Autodesk Inventor part; units mm, degrees
(part 3 of 3)
  line L2014 (13.025, -25.6738) -> (12.925, -25.6738)
  line L2015 (12.9, -26.05) -> (12.8, -26.05)
  line L2016 (12.65, -26.05) -> (12.55, -26.05)
  line L2017 (12.9, -26.35) -> (12.9, -26.05)
  line L2018 (12.8, -26.05) -> (12.8, -26.35)
  line L2019 (12.65, -26.35) -> (12.65, -26.05)
  line L2020 (12.55, -26.05) -> (12.55, -26.35)
  line L2021 (13.4, -26.35) -> (13.4, -26.05)
  line L2022 (13.3, -26.35) -> (13.4, -26.35)
  line L2023 (13.3, -26.05) -> (13.3, -26.35)
  line L2024 (13.15, -26.05) -> (13.05, -26.05)
  line L2025 (13.15, -26.35) -> (13.15, -26.05)
  line L2026 (13.05, -26.05) -> (13.05, -26.35)
  line L2027 (12.8, -26.35) -> (12.9, -26.35)
  line L2028 (12.55, -26.35) -> (12.65, -26.35)
  line L2029 (13.275, -25.9738) -> (13.275, -25.6738)
  line L2030 (13.425, -25.6738) -> (13.425, -25.9738)
  line L2031 (13.525, -25.6738) -> (13.425, -25.6738)
  line L2032 (13.425, -25.9738) -> (13.525, -25.9738)
  line L2033 (13.525, -25.9738) -> (13.525, -25.6738)
  line L2034 (13.675, -25.6738) -> (13.675, -25.9738)
  line L2035 (13.65, -26.05) -> (13.55, -26.05)
  line L2036 (13.775, -25.6738) -> (13.675, -25.6738)
  line L2037 (13.775, -25.9738) -> (13.775, -25.6738)
  line L2038 (13.675, -25.9738) -> (13.775, -25.9738)
  line L2039 (13.4, -26.05) -> (13.3, -26.05)
  line L2040 (13.925, -25.9738) -> (14.025, -25.9738)
  line L2041 (13.925, -25.6738) -> (13.925, -25.9738)
  line L2042 (14.025, -25.9738) -> (14.025, -25.6738)
  line L2043 (14.025, -25.6738) -> (13.925, -25.6738)
  line L2044 (14.425, -25.9738) -> (14.525, -25.9738)
  line L2045 (14.175, -25.9738) -> (14.275, -25.9738)
  line L2046 (14.525, -25.9738) -> (14.525, -25.6738)
  line L2047 (14.275, -25.9738) -> (14.275, -25.6738)
  line L2048 (14.175, -25.6738) -> (14.175, -25.9738)
  line L2049 (14.425, -25.6738) -> (14.425, -25.9738)
  line L2050 (14.525, -25.6738) -> (14.425, -25.6738)
  line L2051 (14.275, -25.6738) -> (14.175, -25.6738)
  line L2052 (14.05, -26.05) -> (14.05, -26.35)
  line L2053 (14.15, -26.05) -> (14.05, -26.05)
  line L2054 (14.05, -26.35) -> (14.15, -26.35)
  line L2055 (14.15, -26.35) -> (14.15, -26.05)
  line L2056 (14.3, -26.05) -> (14.3, -26.35)
  line L2057 (14.4, -26.05) -> (14.3, -26.05)
  line L2058 (14.3, -26.35) -> (14.4, -26.35)
  line L2059 (14.4, -26.35) -> (14.4, -26.05)
  line L2060 (14.55, -26.05) -> (14.55, -26.35)
  line L2061 (13.9, -26.05) -> (13.8, -26.05)
  line L2062 (13.55, -26.05) -> (13.55, -26.35)
  line L2063 (13.55, -26.35) -> (13.65, -26.35)
  line L2064 (13.65, -26.35) -> (13.65, -26.05)
  line L2065 (13.8, -26.05) -> (13.8, -26.35)
  line L2066 (13.9, -26.35) -> (13.9, -26.05)
  line L2067 (13.8, -26.35) -> (13.9, -26.35)
  line L2068 (15.175, -25.6738) -> (15.175, -25.9738)
  line L2069 (15.175, -25.9738) -> (15.275, -25.9738)
  line L2070 (15.275, -25.6738) -> (15.175, -25.6738)
  line L2071 (15.275, -25.9738) -> (15.275, -25.6738)
  line L2072 (15.425, -25.6738) -> (15.425, -25.9738)
  line L2073 (15.525, -25.9738) -> (15.525, -25.6738)
  line L2074 (15.525, -25.6738) -> (15.425, -25.6738)
  line L2075 (15.675, -25.6738) -> (15.675, -25.9738)
  line L2076 (15.775, -25.6738) -> (15.675, -25.6738)
  line L2077 (15.775, -25.9738) -> (15.775, -25.6738)
  line L2078 (15.675, -25.9738) -> (15.775, -25.9738)
  line L2079 (15.425, -25.9738) -> (15.525, -25.9738)
  line L2080 (15.4, -26.05) -> (15.3, -26.05)
  line L2081 (15.65, -26.05) -> (15.55, -26.05)
  line L2082 (15.15, -26.05) -> (15.05, -26.05)
  line L2083 (15.55, -26.35) -> (15.65, -26.35)
  line L2084 (15.65, -26.35) -> (15.65, -26.05)
  line L2085 (15.55, -26.05) -> (15.55, -26.35)
  line L2086 (15.4, -26.35) -> (15.4, -26.05)
  line L2087 (15.3, -26.35) -> (15.4, -26.35)
  line L2088 (15.3, -26.05) -> (15.3, -26.35)
  line L2089 (15.15, -26.35) -> (15.15, -26.05)
  line L2090 (15.05, -26.05) -> (15.05, -26.35)
  line L2091 (15.05, -26.35) -> (15.15, -26.35)
  line L2092 (18.925, -25.6738) -> (18.925, -25.9738)
  line L2093 (18.925, -25.9738) -> (19.025, -25.9738)
  line L2094 (19.025, -25.6738) -> (18.925, -25.6738)
  line L2095 (19.175, -25.6738) -> (19.175, -25.9738)
  line L2096 (19.175, -25.9738) -> (19.275, -25.9738)
  line L2097 (19.275, -25.9738) -> (19.275, -25.6738)
  line L2098 (19.275, -25.6738) -> (19.175, -25.6738)
  line L2099 (19.425, -25.6738) -> (19.425, -25.9738)
  line L2100 (19.425, -25.9738) -> (19.525, -25.9738)
  line L2101 (19.525, -25.9738) -> (19.525, -25.6738)
  line L2102 (19.525, -25.6738) -> (19.425, -25.6738)
  line L2103 (19.025, -25.9738) -> (19.025, -25.6738)
  line L2104 (20.4, -26.05) -> (20.3, -26.05)
  line L2105 (20.425, -25.6738) -> (20.425, -25.9738)
  line L2106 (20.525, -25.9738) -> (20.525, -25.6738)
  line L2107 (20.525, -25.6738) -> (20.425, -25.6738)
  line L2108 (20.425, -25.9738) -> (20.525, -25.9738)
  line L2109 (20.675, -25.6738) -> (20.675, -25.9738)
  line L2110 (20.675, -25.9738) -> (20.775, -25.9738)
  line L2111 (20.775, -25.6738) -> (20.675, -25.6738)
  line L2112 (20.925, -25.6738) -> (20.925, -25.9738)
  line L2113 (21.025, -25.6738) -> (20.925, -25.6738)
  line L2114 (20.925, -25.9738) -> (21.025, -25.9738)
  line L2115 (21.025, -25.9738) -> (21.025, -25.6738)
  line L2116 (20.775, -25.9738) -> (20.775, -25.6738)
  line L2117 (14.9, -26.05) -> (14.8, -26.05)
  line L2118 (14.9, -26.35) -> (14.9, -26.05)
  line L2119 (14.8, -26.35) -> (14.9, -26.35)
  line L2120 (14.8, -26.05) -> (14.8, -26.35)
  line L2121 (14.65, -26.35) -> (14.65, -26.05)
  line L2122 (14.65, -26.05) -> (14.55, -26.05)
  line L2123 (14.55, -26.35) -> (14.65, -26.35)
  line L2124 (14.675, -25.9738) -> (14.775, -25.9738)
  line L2125 (14.925, -25.9738) -> (15.025, -25.9738)
  line L2126 (15.025, -25.9738) -> (15.025, -25.6738)
  line L2127 (15.025, -25.6738) -> (14.925, -25.6738)
  line L2128 (14.925, -25.6738) -> (14.925, -25.9738)
  line L2129 (14.775, -25.9738) -> (14.775, -25.6738)
  line L2130 (14.675, -25.6738) -> (14.675, -25.9738)
  line L2131 (14.775, -25.6738) -> (14.675, -25.6738)
  line L2132 (15.8, -26.05) -> (15.8, -26.35)
  line L2133 (15.8, -26.35) -> (15.9, -26.35)
  line L2134 (15.9, -26.35) -> (15.9, -26.05)
  line L2135 (16.05, -26.05) -> (16.05, -26.35)
  line L2136 (16.05, -26.35) -> (16.15, -26.35)
  line L2137 (16.15, -26.35) -> (16.15, -26.05)
  line L2138 (16.175, -25.9738) -> (16.275, -25.9738)
  line L2139 (16.3, -26.35) -> (16.4, -26.35)
  line L2140 (16.4, -26.05) -> (16.3, -26.05)
  line L2141 (16.4, -26.35) -> (16.4, -26.05)
  line L2142 (16.3, -26.05) -> (16.3, -26.35)
  line L2143 (16.425, -25.9738) -> (16.525, -25.9738)
  line L2144 (16.525, -25.9738) -> (16.525, -25.6738)
  line L2145 (16.425, -25.6738) -> (16.425, -25.9738)
  line L2146 (16.525, -25.6738) -> (16.425, -25.6738)
  line L2147 (15.9, -26.05) -> (15.8, -26.05)
  line L2148 (16.025, -25.9738) -> (16.025, -25.6738)
  line L2149 (15.925, -25.9738) -> (16.025, -25.9738)
  line L2150 (16.025, -25.6738) -> (15.925, -25.6738)
  line L2151 (16.175, -25.6738) -> (16.175, -25.9738)
  line L2152 (16.275, -25.9738) -> (16.275, -25.6738)
  line L2153 (16.275, -25.6738) -> (16.175, -25.6738)
  line L2154 (16.15, -26.05) -> (16.05, -26.05)
  line L2155 (15.925, -25.6738) -> (15.925, -25.9738)
  line L2156 (16.55, -26.05) -> (16.55, -26.35)
  line L2157 (16.65, -26.05) -> (16.55, -26.05)
  line L2158 (16.55, -26.35) -> (16.65, -26.35)
  line L2159 (16.65, -26.35) -> (16.65, -26.05)
  line L2160 (16.8, -26.05) -> (16.8, -26.35)
  line L2161 (16.8, -26.35) -> (16.9, -26.35)
  line L2162 (16.9, -26.35) -> (16.9, -26.05)
  line L2163 (16.9, -26.05) -> (16.8, -26.05)
  line L2164 (16.675, -25.9738) -> (16.775, -25.9738)
  line L2165 (16.775, -25.9738) -> (16.775, -25.6738)
  line L2166 (16.775, -25.6738) -> (16.675, -25.6738)
  line L2167 (16.675, -25.6738) -> (16.675, -25.9738)
  line L2168 (17.15, -26.05) -> (17.05, -26.05)
  line L2169 (16.925, -25.6738) -> (16.925, -25.9738)
  line L2170 (17.025, -25.9738) -> (17.025, -25.6738)
  line L2171 (17.025, -25.6738) -> (16.925, -25.6738)
  line L2172 (17.175, -25.9738) -> (17.275, -25.9738)
  line L2173 (17.175, -25.6738) -> (17.175, -25.9738)
  line L2174 (17.275, -25.9738) -> (17.275, -25.6738)
  line L2175 (17.275, -25.6738) -> (17.175, -25.6738)
  line L2176 (16.925, -25.9738) -> (17.025, -25.9738)
  line L2177 (17.675, -25.9738) -> (17.775, -25.9738)
  line L2178 (17.425, -25.9738) -> (17.525, -25.9738)
  line L2179 (17.425, -25.6738) -> (17.425, -25.9738)
  line L2180 (17.525, -25.6738) -> (17.425, -25.6738)
  line L2181 (17.525, -25.9738) -> (17.525, -25.6738)
  line L2182 (17.675, -25.6738) -> (17.675, -25.9738)
  line L2183 (17.775, -25.6738) -> (17.675, -25.6738)
  line L2184 (17.775, -25.9738) -> (17.775, -25.6738)
  line L2185 (17.925, -25.9738) -> (18.025, -25.9738)
  line L2186 (18.175, -25.9738) -> (18.275, -25.9738)
  line L2187 (18.275, -25.6738) -> (18.175, -25.6738)
  line L2188 (18.275, -25.9738) -> (18.275, -25.6738)
  line L2189 (18.175, -25.6738) -> (18.175, -25.9738)
  line L2190 (18.025, -25.9738) -> (18.025, -25.6738)
  line L2191 (18.025, -25.6738) -> (17.925, -25.6738)
  line L2192 (17.925, -25.6738) -> (17.925, -25.9738)
  line L2193 (17.4, -26.05) -> (17.3, -26.05)
  line L2194 (17.05, -26.35) -> (17.15, -26.35)
  line L2195 (17.05, -26.05) -> (17.05, -26.35)
  line L2196 (17.15, -26.35) -> (17.15, -26.05)
  line L2197 (17.65, -26.05) -> (17.55, -26.05)
  line L2198 (17.3, -26.05) -> (17.3, -26.35)
  line L2199 (17.3, -26.35) -> (17.4, -26.35)
  line L2200 (17.55, -26.05) -> (17.55, -26.35)
  line L2201 (17.65, -26.35) -> (17.65, -26.05)
  line L2202 (17.55, -26.35) -> (17.65, -26.35)
  line L2203 (17.8, -26.05) -> (17.8, -26.35)
  line L2204 (17.4, -26.35) -> (17.4, -26.05)
  line L2205 (17.9, -26.05) -> (17.8, -26.05)
  line L2206 (17.8, -26.35) -> (17.9, -26.35)
  line L2207 (18.15, -26.05) -> (18.05, -26.05)
  line L2208 (17.9, -26.35) -> (17.9, -26.05)
  line L2209 (18.4, -26.05) -> (18.3, -26.05)
  line L2210 (18.05, -26.05) -> (18.05, -26.35)
  line L2211 (18.05, -26.35) -> (18.15, -26.35)
  line L2212 (18.15, -26.35) -> (18.15, -26.05)
  line L2213 (18.3, -26.05) -> (18.3, -26.35)
  line L2214 (18.3, -26.35) -> (18.4, -26.35)
  line L2215 (18.4, -26.35) -> (18.4, -26.05)
  line L2216 (19.05, -26.05) -> (19.05, -26.35)
  line L2217 (19.15, -26.35) -> (19.15, -26.05)
  line L2218 (19.05, -26.35) -> (19.15, -26.35)
  line L2219 (19.3, -26.05) -> (19.3, -26.35)
  line L2220 (19.3, -26.35) -> (19.4, -26.35)
  line L2221 (19.4, -26.05) -> (19.3, -26.05)
  line L2222 (19.15, -26.05) -> (19.05, -26.05)
  line L2223 (18.55, -26.05) -> (18.55, -26.35)
  line L2224 (18.55, -26.35) -> (18.65, -26.35)
  line L2225 (18.65, -26.35) -> (18.65, -26.05)
  line L2226 (18.9, -26.05) -> (18.8, -26.05)
  line L2227 (18.8, -26.05) -> (18.8, -26.35)
  line L2228 (18.9, -26.35) -> (18.9, -26.05)
  line L2229 (18.8, -26.35) -> (18.9, -26.35)
  line L2230 (18.425, -25.9738) -> (18.525, -25.9738)
  line L2231 (18.675, -25.9738) -> (18.775, -25.9738)
  line L2232 (18.775, -25.6738) -> (18.675, -25.6738)
  line L2233 (18.675, -25.6738) -> (18.675, -25.9738)
  line L2234 (18.65, -26.05) -> (18.55, -26.05)
  line L2235 (18.525, -25.9738) -> (18.525, -25.6738)
  line L2236 (18.425, -25.6738) -> (18.425, -25.9738)
  line L2237 (18.525, -25.6738) -> (18.425, -25.6738)
  line L2238 (18.775, -25.9738) -> (18.775, -25.6738)
  line L2239 (19.65, -26.05) -> (19.55, -26.05)
  line L2240 (19.4, -26.35) -> (19.4, -26.05)
  line L2241 (19.55, -26.05) -> (19.55, -26.35)
  line L2242 (19.55, -26.35) -> (19.65, -26.35)
  line L2243 (19.65, -26.35) -> (19.65, -26.05)
  line L2244 (19.9, -26.05) -> (19.8, -26.05)
  line L2245 (19.8, -26.05) -> (19.8, -26.35)
  line L2246 (19.9, -26.35) -> (19.9, -26.05)
  line L2247 (19.8, -26.35) -> (19.9, -26.35)
  line L2248 (20.05, -26.05) -> (20.05, -26.35)
  line L2249 (20.15, -26.05) -> (20.05, -26.05)
  line L2250 (20.05, -26.35) -> (20.15, -26.35)
  line L2251 (20.15, -26.35) -> (20.15, -26.05)
  line L2252 (20.3, -26.05) -> (20.3, -26.35)
  line L2253 (20.4, -26.35) -> (20.4, -26.05)
  line L2254 (20.3, -26.35) -> (20.4, -26.35)
  line L2255 (20.55, -26.05) -> (20.55, -26.35)
  line L2256 (20.65, -26.05) -> (20.55, -26.05)
  line L2257 (20.55, -26.35) -> (20.65, -26.35)
  line L2258 (20.65, -26.35) -> (20.65, -26.05)
  line L2259 (20.8, -26.05) -> (20.8, -26.35)
  line L2260 (20.9, -26.35) -> (20.9, -26.05)
  line L2261 (20.8, -26.35) -> (20.9, -26.35)
  line L2262 (20.9, -26.05) -> (20.8, -26.05)
  line L2263 (19.675, -25.9738) -> (19.775, -25.9738)
  line L2264 (20.275, -25.9738) -> (20.275, -25.6738)
  line L2265 (20.175, -25.9738) -> (20.275, -25.9738)
  line L2266 (20.175, -25.6738) -> (20.175, -25.9738)
  line L2267 (20.025, -25.9738) -> (20.025, -25.6738)
  line L2268 (19.925, -25.9738) -> (20.025, -25.9738)
  line L2269 (19.925, -25.6738) -> (19.925, -25.9738)
  line L2270 (20.025, -25.6738) -> (19.925, -25.6738)
  line L2271 (19.775, -25.9738) -> (19.775, -25.6738)
  line L2272 (19.675, -25.6738) -> (19.675, -25.9738)
  line L2273 (19.775, -25.6738) -> (19.675, -25.6738)
  line L2274 (20.275, -25.6738) -> (20.175, -25.6738)
  point P0 (0, 0)
  dimension "d57" = 0.1
  dimension "d58" = 0.3
  dimension "d59" = 3.25
  dimension "d60" = 1.9
  dimension "d63" = 0.25
  dimension "d68" = 0.3
  dimension "d69" = 0.1
  dimension "d70" = 0.125
  dimension "d71" = 0.0762
  dimension "d74" = 0.25
  dimension "d83" = 21.6
  dimension "d90" = 360
  constraints: 4546 end point, 6 horizontal, 4 parallel, 2 perpendicular, 6801 other
  measures "d57" distance of L2.end L1.end
  measures "d58" distance of L1.end L0.end
  measures "d59" distance between parallel lines of L4 L3
  measures "d60" distance between parallel lines of L5 L0
  measures "d63" distance of L0.start L6.start
  measures "d68" distance of L288.end L286.start
  measures "d69" distance of L287.end L288.end
  measures "d70" distance between parallel lines of L289 L3
  measures "d71" distance between parallel lines of L286 L2
  measures "d74" distance of L287.end L290.end
  measures "d83" distance of L0.start L570.start
extrude "Extrusion4" add sketch "Sketch8" along normal blind 0.05
equation "\"d68\" = d58"
equation "\"d69\" = d57"
equation "\"d70\" = 0.5 * d63"
body "Solid1"
